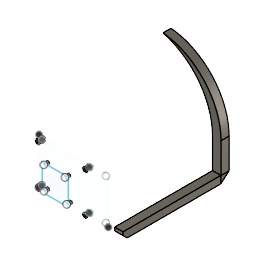
case (Autodesk Fusion 360 design; units mm, degrees)
Autodesk Fusion 360 part; units mm, degrees
sketch "Sketch2" plane through (0, 0, 0) normal (0, 1, 0) x (1, 0, 0)
  line L0 (3, 0) -> (82, 0)
  line L1 (85, -3) -> (85, -53)
  line L2 (82, -56) -> (3, -56)
  line L3 (0, -53) -> (0, -3)
  arc A0 (0, -53) -> (3, -56) centre (3, -53) ccw
  arc A1 (82, -56) -> (85, -53) centre (82, -53) ccw
  arc A2 (85, -3) -> (82, 0) centre (82, -3) ccw
  arc A3 (3, 0) -> (0, -3) centre (3, -3) ccw
  circle A4 centre (61.5, -52.1984) radius 3
  circle A5 centre (3.5, -52.5) radius 3
  circle A6 centre (3.5, -3.5) radius 3
  circle A7 centre (61.5, -3.5) radius 3
  point P0 (85, 0)
  point P1 (0, -56)
  point P2 (3.5, -52.5)
  point P3 (3.5, -3.5)
  point P4 (61.5, -52.1984)
  point P5 (61.5, -3.5)
  dimension "d3" = 85
  dimension "d4" = 56
  dimension "d5" = 3
  dimension "d6" = 3
  dimension "d7" = 3.5
  dimension "d8" = 3.5
  dimension "d9" = 3.5
  dimension "d10" = 3.5
  dimension "d11" = 23.5
  dimension "d12" = 6
  dimension "d13" = 6
  dimension "d14" = 6
  dimension "d15" = 6
  constraint horizontal L0
  constraint vertical L1
  constraint horizontal L2
  constraint vertical L3
  constraint coincident P1 L2
  constraint coincident P1 L3
  constraint tangent L2 A0
  constraint tangent L3 A0
  constraint tangent L1 A1
  constraint tangent L2 A1
  constraint equal A0 A1
  constraint coincident P0 L0
  constraint coincident P0 L1
  constraint tangent L0 A2
  constraint tangent L1 A2
  constraint equal A0 A2
  constraint coincident origin L0
  constraint coincident origin L3
  constraint tangent L0 A3
  constraint tangent L3 A3
  constraint coincident P4 A4.centre
  constraint coincident P2 A5.centre
  constraint coincident P3 A6.centre
  constraint coincident P5 A7.centre
  measures "d3" distance of origin P0
  measures "d4" distance of origin P1
  measures "d5" radius of A0
  measures "d6" radius of A3
  measures "d7" distance of L2 P2
  measures "d8" distance of L3 P2
  measures "d9" distance of L0 P3
  measures "d10" distance of L3 P3
  measures "d11" distance of L1 P4
  measures "d12" diameter of A4
  measures "d13" diameter of A5
  measures "d14" diameter of A6
  measures "d15" diameter of A7
extrude "Extrude2" add sketch "Sketch2" against normal blind 5 contours A4 | A5 | A6 | A7 makes body 1 at (6.4963, -3.3333, 3.6495) makes body 2 at (64.4963, -3.3333, 3.6495) makes body 3 at (6.4963, -3.3333, 52.6495) makes body 4 at (58.5149, -3.3333, 52.4971)
hole "Hole1" at (3.5, 0, 52.5) direction (0, -1, 0) diameter 2.7 depth 10 tip angle 118 bodies 3
hole "Hole2" at (3.5, 0, 3.5) direction (0, -1, 0) diameter 2.7 depth 10 tip angle 118 bodies 1
hole "Hole3" at (61.5, 0, 52.1984) direction (0, -1, 0) diameter 2.7 depth 10 tip angle 118 bodies 4
hole "Hole4" at (61.5, 0, 3.5) direction (0, -1, 0) diameter 2.7 depth 10 tip angle 118 bodies 2
ref_plane "WorkPlane1" through (42.5, -15, 28) normal (0, 1, 0) x (1, 0, 0)
sketch "Sketch3" plane through (0, -15, 0) normal (0, 1, 0) x (1, 0, 0)
  line L0 (18.8859, -43.7341) -> (50.8859, -43.7341)
  line L1 (50.8859, -43.7341) -> (50.8859, -11.7341)
  line L2 (50.8859, -11.7341) -> (18.8859, -11.7341)
  line L3 (18.8859, -11.7341) -> (18.8859, -43.7341)
  circle A0 centre (20.8859, -41.7341) radius 2
  circle A1 centre (46.7326, -41.309) radius 2
  circle A2 centre (20.8859, -13.7341) radius 2
  circle A3 centre (20.8859, -41.7341) radius 1
  circle A4 centre (20.8859, -13.7341) radius 1
  circle A5 centre (46.7326, -41.309) radius 1
  circle A6 centre (48.8859, -13.7341) radius 2
  circle A7 centre (48.8859, -13.7341) radius 1
  dimension "d31" = 32
  dimension "d32" = 32
  dimension "d36" = 4
  dimension "d37" = 2
  dimension "d38" = 2
  dimension "d39" = 4
  dimension "d40" = 4
  dimension "d41" = 2
  dimension "d42" = 2
  dimension "d43" = 2
  dimension "d46" = 2
  dimension "d47" = 2
  dimension "d48" = 4
  dimension "d49" = 2
  dimension "d50" = 2
  dimension "d51" = 2
  constraint horizontal L0
  constraint vertical L1
  constraint horizontal L2
  constraint vertical L3
  constraint concentric A0 A3
  constraint concentric A2 A4
  constraint concentric A1 A5
  constraint concentric A6 A7
  measures "d31" distance of L0.start L0.end
  measures "d32" distance of L0.start L2.end
  measures "d36" diameter of A0
  measures "d37" distance of L0 A0.centre
  measures "d38" distance of L3 A0.centre
  measures "d39" diameter of A1
  measures "d40" diameter of A2
  measures "d41" diameter of A3
  measures "d42" diameter of A4
  measures "d43" diameter of A5
  measures "d46" distance of L2 A2.centre
  measures "d47" distance of L3 A2.centre
  measures "d48" diameter of A6
  measures "d49" distance of L1 A6.centre
  measures "d50" distance of L2 A6.centre
  measures "d51" diameter of A7
extrude "Extrude3" add sketch "Sketch3" along normal blind 5 separate body contours A0 | A2 | A6 | A1 makes body 5 at (22.8759, -11.6667, 41.535) makes body 6 at (22.8759, -11.6667, 13.535) makes body 7 at (48.3268, -11.6667, 40.1014) makes body 8 at (50.8759, -11.6667, 13.535)
ref_plane "WorkPlane2" through (42.5, 114, 28) normal (0, 1, 0) x (1, 0, 0)
sketch "Sketch5" plane through (0, 114, 0) normal (0, 1, 0) x (1, 0, 0)
  line L0 (109.2491, -47.1152) -> (98.7423, -47.1152)
  line L1 (98.7423, -47.1152) -> (98.7423, -10.147)
  line L2 (98.7423, -10.147) -> (109.2491, -10.147)
  line L3 (109.2491, -10.147) -> (109.2491, -47.1152)
  arc A0 (38.0127, -126.0957) -> (109.2491, -47.1152) centre (29.8477, -47.1152) ccw
  arc A1 (38.0127, -126.0957) -> (98.7423, -47.1152) centre (17.0194, -47.1152) ccw
  constraint horizontal L0
  constraint vertical L1
  constraint horizontal L2
  constraint vertical L3
  constraint tangent L3 A0
  constraint tangent L1 A1
extrude "Extrude4" add sketch "Sketch5" along normal blind 10 separate body makes body 9
sketch "Sketch6" plane through (0, 0, 0) normal (0, 1, 0) x (1, 0, 0)
  circle A0 centre (61.5, -52.1984) radius 1.35
  circle A1 centre (3.5, -52.5) radius 1.35
  circle A2 centre (3.5, -3.5) radius 1.35
  circle A3 centre (61.5, -3.5) radius 1.35
extrude "Extrude5" add sketch "Sketch6" along normal blind -33 and the other way blind -25 separate body makes body 10 at (60.1567, -13.6667, 52.3328) makes body 11 at (62.8483, -13.6667, 3.5673) makes body 12 at (2.1567, -13.6667, 52.6344) makes body 13 at (4.8483, -13.6667, 3.5673)
extrude "Extrude6" add sketch "Sketch3" along normal blind 28 and the other way blind 14 separate body contours A3 | A4 | A5 | A7 makes body 14 at (21.866, 3.6667, 41.9323) makes body 15 at (21.8809, 3.6667, 13.8337) makes body 16 at (45.8543, 3.6667, 41.7873) makes body 17 at (48.2242, 3.6667, 14.4839)
extrude "Extrude7" add sketch "Sketch2" along normal blind 75 separate body makes body 18
sketch "Sketch7" plane through (0, 124, 0) normal (0, 1, 0) x (-1, 0, 0)
  arc A0 (-38.0127, 126.0957) -> (-109.2491, 47.1152) centre (-29.8477, 47.1152) ccw
  line L0 (-109.2491, 47.1152) -> (-109.2491, 10.147)
  line L1 (-109.2491, 10.147) -> (-98.7423, 10.147)
  line L2 (-98.7423, 10.147) -> (-98.7423, 47.1152)
  arc A1 (-38.0127, 126.0957) -> (-98.7423, 47.1152) centre (-17.0194, 47.1152) ccw
  arc A2 (-98.7423, 10.147) -> (-60, -70) centre (3.5297, 10.147) ccw
  line L3 (-60, -70) -> (61.736, -70)
  line L4 (61.736, -70) -> (61.736, 124.8737)
  line L5 (61.736, 124.8737) -> (-38.0127, 126.0957)
  constraint coincident L1.end L2.start
  constraint tangent L2 A2
  constraint perpendicular L2 L3
  constraint perpendicular L3 L4
  constraint coincident A0.start A1.start
extrude "Extrude8" add sketch "Sketch7" against normal blind 50 separate body contours L2 A1 A2 L3 L4 L5 makes body 19
sketch "Sketch8" plane through (0, 114, 0) normal (0, -1, 0) x (1, 0, 0)
  arc A0 (109.2491, 47.1152) -> (38.0127, 126.0957) centre (29.8477, 47.1152) ccw
  arc A1 (98.7423, 47.1152) -> (38.0127, 126.0957) centre (17.0194, 47.1152) ccw
  line L0 (98.7423, 47.1152) -> (98.7423, 10.147)
  line L1 (98.7423, 10.147) -> (109.2491, 10.147)
  line L2 (109.2491, 10.147) -> (109.2491, 47.1152)
  line L3 (98.7423, 11.3094) -> (109.0078, 11.3094)
  line L4 (109.0078, 11.3094) -> (109.0078, 1.0525)
  line L5 (109.0078, 1.0525) -> (98.7423, 1.0525)
  line L6 (98.7423, 1.0525) -> (98.7423, 11.3094)
  constraint horizontal L3
  constraint vertical L4
  constraint horizontal L5
  constraint vertical L6
  constraint coincident L0 L3.start
extrude "Extrude9" add sketch "Sketch8" along normal blind 120 separate body contours L1 L4 L5 L6 makes body 20
loft "Loft1" add section 1 face at (105.586, 114, 7.1155) section 2 face at (102.2446, 117.3333, 10.147) on bodies 9 20 bodies 9 20
chamfer "Chamfer1" distance 5 angle 45 1 edges at (103.8751, -6, 1.0525) on bodies 9
equation "d13 = d12"
equation "d14 = d12"
equation "d15 = d12"
